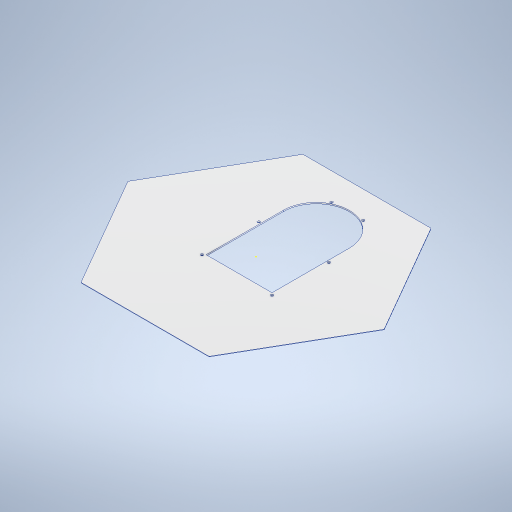
# Autodesk Inventor part: AEON.AluminiumFrame
Saved by Autodesk Inventor 2023.2 (Build 272271000, 271)
## iProperties
Created: 2022-07-15
Part Number: AEON.AluminiumFrame
Material: Generic
Document SubType Name: Modeling
Designer: delh
Mass: 169.93 g
Surface Area: 2007.75 cm^2
Volume: 169.93 cm^3
Density: 1 g/cm^3
Appearance: Default
Author: delh
Autodesk Inventor part; units mm, degrees
ref_plane "YZ Plane" through (0, 0, 0) normal (1, 0, 0) x (0, 1, 0)
ref_plane "XZ Plane" through (0, 0, 0) normal (0, 1, 0) x (-1, 0, 0)
ref_plane "XY Plane" through (0, 0, 0) normal (0, 0, 1) x (1, 0, 0)
sketch "Sketch1" plane through (0, 0, 0) normal (0, 0, 1) x (1, 0, 0)
  line L0 (212.4649, 0) -> (106.2324, -184)
  line L1 (106.2324, -184) -> (-106.2324, -184)
  line L2 (-106.2324, -184) -> (-212.4649, 0)
  line L3 (-212.4649, 0) -> (-106.2324, 184)
  line L4 (-106.2324, 184) -> (106.2324, 184)
  line L5 (106.2324, 184) -> (212.4649, 0)
  point P0 (0, 0)
  point P1 (0, 0)
  dimension "d0" = 368
  constraints: 12 end point, 1 coincident, 13 other
  measures "d0" distance between parallel lines of L1 L4
extrude "Extrusion1" add sketch "Sketch1" along normal blind 2
sketch "Sketch7" plane through (0, 0, 0) normal (0, 0, -1) x (-1, 0, 0)
  line L0 (-66.5995, 87.3368) -> (-66.5995, -40)
  line L1 (41.5995, 87.3368) -> (41.5995, -40)
  line L2 (-66.5995, -40) -> (41.5995, -40)
  arc A0 (41.5995, 87.3368) -> (-66.5995, 87.3368) centre (-12.5, 87.3368) ccw
  point P0 (0, 0)
  constraints: 6 end point, 2 point on circle, 1 centre point
extrude "Extrusion5" cut sketch "Sketch7" against normal blind 10
sketch "Sketch8" plane through (0, 0, 0) normal (0, 0, -1) x (-1, 0, 0)
  line L0 (-191.6803, 0) -> (-95.8401, 166)
  line L1 (-95.8401, 166) -> (96.1778, 166)
  line L2 (96.1778, 166) -> (191.5124, -0.2908)
  line L3 (191.5124, -0.2908) -> (95.8401, -166)
  line L4 (95.8401, -166) -> (-95.8401, -166)
  line L5 (-95.8401, -166) -> (-191.6803, 0)
  line L6 (-106.2324, -184) -> (-212.4649, 0) projected
  line L7 (-106.2324, -184) -> (-212.4649, 0)
  line L8 (106.2324, -184) -> (-106.2324, -184) projected
  line L9 (-106.2324, -184) -> (106.2324, -184)
  line L10 (212.4649, 0) -> (106.2324, -184) projected
  line L11 (106.2324, -184) -> (212.2788, -0.3224)
  line L12 (106.2324, 184) -> (212.4649, 0) projected
  line L13 (212.2788, -0.3224) -> (106.6066, 184)
  line L14 (-106.2324, 184) -> (106.2324, 184) projected
  line L15 (-106.2324, 184) -> (297.9127, 184)
  line L16 (-212.4649, 0) -> (-106.2324, 184) projected
  line L17 (-212.4649, 0) -> (-106.2324, 184)
  line L18 (-106.2324, 184) -> (106.2324, 184) projected
  point P0 (0, 0)
  dimension "d25" = 18
  dimension "d26" = 18
  dimension "d27" = 18
  dimension "d28" = 18
  dimension "d29" = 18
  dimension "d30" = 18
  constraints: 24 end point, 8 point on line, 2 parallel, 1 collinear, 1 equal length
  measures "d25" distance between parallel lines of L5 L7
  measures "d26" distance between parallel lines of L4 L9
  measures "d27" distance between parallel lines of L0 L16
  measures "d28" distance between parallel lines of L15 L1
  measures "d29" distance between parallel lines of L11 L3
  measures "d30" distance between parallel lines of L13 L2
extrude "Extrusion6" cut sketch "Sketch8" against normal blind 1.25 contours L6 L16 L14 L12 L13 L10 L8 | L13 L12 L10
fillet "Fillet1" radius 5 6 edges at (-96.1778, 166, 0.625) (-191.5124, -0.2908, 0.625) (-95.8401, -166, 0.625) (95.8401, -166, 0.625) (191.6803, 0, 0.625) (95.8401, 166, 0.625)
sketch "Sketch10" plane through (0, 0, 0) normal (0, 0, -1) x (-1, 0, 0)
  circle A0 centre (13.7082, 139) radius 0.7835 projected
  circle A1 centre (45.5995, 50.2789) radius 0.7835 projected
  circle A2 centre (45.5995, -44) radius 0.7835 projected
  circle A3 centre (-70.5995, -44) radius 0.7835 projected
  circle A4 centre (-70.5995, 50.2789) radius 0.7835 projected
  circle A5 centre (-38.7082, 139) radius 0.7835 projected
  point P0 (0, 0)
extrude "Extrusion8" cut sketch "Sketch10" against normal blind 10
sketch "Sketch11" plane through (0, 0, 0) normal (0, 0, -1) x (-1, 0, 0)
  point P0 (0, 0)
sketch "Sketch12" plane through (0, 0, 2) normal (0, 0, 1) x (1, 0, 0)
  arc A0 (66.5995, 87.3368) -> (-41.5995, 87.3368) centre (12.5, 87.3368) ccw projected
  line L0 (-41.5995, -40) -> (-41.5995, 87.3368) projected
  line L1 (66.5995, 87.3368) -> (66.5995, -40) projected
  line L2 (66.5995, -40) -> (-41.5995, -40) projected
  arc A1 (67.0995, 87.3368) -> (-42.0995, 87.3368) centre (12.5, 87.3368) ccw
  line L3 (67.0995, 87.3368) -> (67.0995, -40.5)
  line L4 (67.0995, -40.5) -> (-42.0995, -40.5)
  line L5 (-42.0995, -40.5) -> (-42.0995, 87.3368)
  point P0 (0, 0)
  dimension "d35" = 0.5
  constraints: 6 end point, 2 point on circle, 1 centre point, 3 other
  measures "d35" distance between parallel lines of L0 L5
extrude "Extrusion9" cut sketch "Sketch12" against normal blind 10 contours L1 L2 L0 A0 | L3 L4 L5 A1
sketch "Sketch13" plane through (0, 0, 2) normal (0, 0, 1) x (1, 0, 0)
  circle A0 centre (-13.7082, 139) radius 0.7835 projected
  circle A1 centre (38.7082, 139) radius 0.7835 projected
  circle A2 centre (70.5995, 50.2789) radius 0.7835 projected
  circle A3 centre (-45.5995, 50.2789) radius 0.7835 projected
  circle A4 centre (70.5995, -44) radius 0.7835 projected
  circle A5 centre (-45.5995, -44) radius 0.7835 projected
  point P0 (0, 0)
hole "Hole1" at (-45.5995, -44, 2) at (70.5995, -44, 2) at (70.5995, 50.2789, 2) at (-13.7082, 139, 2) at (38.7082, 139, 2) at (-45.5995, 50.2789, 2) direction (0, 0, -1) diameter 2.4 depth 3 tip angle 118 countersink diameter 4.4 countersink angle 90 clearance for "Countersunk Flat Head Screw ISO 2009/7046" size "M2" standard "ISO"
equation "\"d26\" = d25"
equation "\"d27\" = d25"
equation "\"d28\" = d25"
equation "\"d29\" = d25"
equation "\"d30\" = d25"
body "Solid1"
